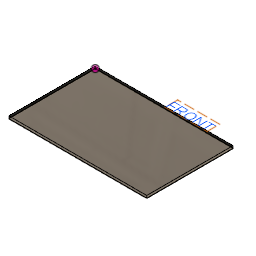
Irrigation unit - Main box (side mounted) v18 (Autodesk Fusion 360 archive; units mm, degrees)
design "_ Solar panel (ZW 110x69)"
Autodesk Fusion 360 part; units mm, degrees
sketch "Sketch1" plane through (0, 0, 0) normal (0, 0, 1) x (1, 0, 0)
  line L0 (0, 0) -> (110, 0)
  line L1 (110, 0) -> (110, -69)
  line L2 (110, -69) -> (0, -69)
  line L3 (0, -69) -> (0, 0)
  line L4 (54.46, 1.171) -> (87.8779, 1.171) construction
  line L5 (87.8779, 1.171) -> (87.8779, 11.171) construction
  line L6 (87.8779, 11.171) -> (54.46, 11.171) construction
  line L7 (54.46, 11.171) -> (54.46, 1.171) construction
  dimension "d1" = 69
  dimension "d2" = 110
extrude "Extrude1" add sketch "Sketch1" along normal blind 2

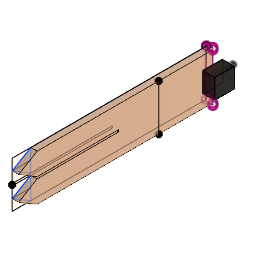
design "_ humidity sensor"
Autodesk Fusion 360 part; units mm, degrees
sketch "Sketch1" plane through (0, 0, 0) normal (1, 0, 0) x (0, 0, -1)
  line L0 (0, 0) -> (23, 0)
  line L1 (23, 0) -> (23, -97)
  line L2 (23, -97) -> (0, -97)
  line L3 (0, -97) -> (0, 0)
  line L4 (11, -47) -> (12, -47)
  line L5 (12, -47) -> (12, -97)
  line L6 (12, -97) -> (11, -97)
  line L7 (11, -97) -> (11, -47)
  line L8 (0, -87.7196) -> (11, -87.7196)
  line L9 (12, -87.7196) -> (23, -87.7196)
  line L10 (5.5, -87.7196) -> (5.5, -97)
  line L11 (17.5, -87.7196) -> (17.5, -97)
  line L12 (17.5, -97) -> (12, -87.7196)
  line L13 (17.5, -97) -> (23, -87.7196)
  line L14 (5.5, -97) -> (0, -87.7196)
  line L15 (5.5, -97) -> (11, -87.7196)
  point P0 (11.5, -97)
  dimension "d46" = 97
  dimension "d47" = 23
  dimension "d48" = 1
  dimension "d49" = 50
  constraint horizontal L0
  constraint vertical L1
  constraint horizontal L2
  constraint vertical L3
  constraint coincident L0.start L3.end
  constraint horizontal L4
  constraint vertical L5
  constraint horizontal L6
  constraint vertical L7
  constraint collinear L2 L6
  constraint midpoint L6 P0
  constraint midpoint L2 P0
  constraint coincident L3 L8.start
  constraint coincident L7 L8.end
  constraint perpendicular L7 L8
  constraint coincident L5 L9.start
  constraint coincident L1 L9.end
  constraint perpendicular L1 L9
  constraint midpoint L8 L10.start
  constraint coincident L2 L10.end
  constraint perpendicular L2 L10
  constraint midpoint L9 L11.start
  constraint perpendicular L9 L11
  constraint collinear L8 L9
  constraint parallel L13 L15
  measures "d46" distance of L0.start L2.end
  measures "d47" distance of L0.start L0.end
  measures "d48" distance of L4.start L4.end
  measures "d49" distance of L4.start L6.end
extrude "Extrude1" add sketch "Sketch1" along normal blind 3.2 contours L0 L1 L3 L4 L5 L7 L8 L9 | L8 L10 L14 | L9 L11 L13 | L8 L10 L15 | L9 L11 L12 makes body 1
ref_plane "WorkPlane1" through (3.2, -48.5, -11.5) normal (1, 0, 0) x (0, 0, -1)
sketch "Sketch2" plane through (3.2, -30, -10) normal (1, 0, 0) x (0, 0, -1)
  line L0 (-3.5, 25) -> (6.5, 25)
  line L1 (6.5, 25) -> (6.5, 35)
  line L2 (6.5, 35) -> (-3.5, 35)
  line L3 (-3.5, 35) -> (-3.5, 25)
  line L4 (13, 30) -> (-10, 30)
  line L5 (1.5, 30) -> (1.5, 40) construction
  dimension "d60" = 10
  dimension "d61" = 10
  dimension "d1" = 5
  constraint horizontal L0
  constraint vertical L1
  constraint horizontal L2
  constraint vertical L3
  constraint midpoint L4 L5.start
  constraint perpendicular L4 L5
  constraint midpoint L2 L5
  measures "d60" distance of L0.start L0.end
  measures "d61" distance of L0.start L2.end
  measures "d1" distance of L2 L4
extrude "Extrude2" add sketch "Sketch2" along normal blind 6 separate body makes body 2
sketch "used for creating hole in the outer box" plane through (0, 0, 0) normal (0, 1, 0) x (-1, 0, 0)
  line L0 (0, -23) -> (0, 0)
  line L1 (0, 0) -> (-3.2, 0)
  line L2 (-3.2, 0) -> (-3.2, -23)
  line L3 (-3.2, -23) -> (0, -23)
  line L4 (-3.2, -24) -> (0.5, -24)
  line L5 (0.5, -24) -> (0.5, 1)
  line L6 (0.5, 1) -> (-3.2, 1)
  line L7 (-3.2, 1) -> (-3.2, -24)
  line L8 (0, 0) -> (0, -23)
  dimension "d181" = 1
  dimension "d182" = 1
  dimension "d2" = 0.5
  constraint horizontal L4
  constraint vertical L5
  constraint horizontal L6
  constraint vertical L7
  constraint collinear L2 L7
  measures "d181" distance of L3 L4
  measures "d182" distance of L1 L6
  measures "d2" distance of L0 L5
sketch "Sketch6" plane through (3.2, 0, 0) normal (1, 0, 0) x (0, 1, 0)
  line L0 (-87.7196, 0) -> (-97, -5.5)
  line L1 (-97, -5.5) -> (-87.7196, -11)
  line L2 (-87.7196, -11) -> (-47, -11)
  line L3 (-47, -11) -> (-47, -12)
  line L4 (-47, -12) -> (-87.7196, -12)
  line L5 (-87.7196, -12) -> (-97, -17.5)
  line L6 (-97, -17.5) -> (-87.7196, -23)
  line L7 (-87.7196, -23) -> (0, -23)
  line L8 (0, -23) -> (0, 0)
  line L9 (0, 0) -> (-87.7196, 0)
  line L10 (-27, 0) -> (-27, -23)
  line L11 (0, 1) -> (0, -24)
  dimension "d3" = 27
  constraint coincident L9 L10.start
  constraint coincident L7 L10.end
  constraint perpendicular L7 L10
  measures "d3" distance of L10 L11
